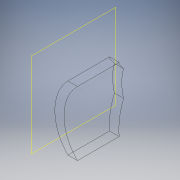
# Autodesk Inventor part: 14mm_radius_mold_with_crystal_skull
Saved by Autodesk Inventor 2018 (Build 220112000, 112)
## iProperties
Created: 2018-06-11
Part Number: 14mm_radius_mold_with_crystal_skull
Material: Generic
Document SubType Name: Modeling
Designer: McCormick Lab
Density: 1 g/cm^3
Appearance: Default
Author: McCormick Lab
Autodesk Inventor part; units mm, degrees
ref_plane "YZ Plane" through (0, 0, 0) normal (1, 0, 0) x (0, 1, 0)
ref_plane "XZ Plane" through (0, 0, 0) normal (0, 1, 0) x (-1, 0, 0)
ref_plane "XY Plane" through (0, 0, 0) normal (0, 0, 1) x (1, 0, 0)
sketch "Sketch1" plane through (0, 0, 0) normal (0, 1, 0) x (-1, 0, 0)
  arc A0 (0, -7) -> (0, 7) centre (0, 0) ccw
  line L0 (0, 7) -> (0, -7)
  dimension "d0" = 14
  constraints: 2 end point, 2 point on circle, 1 centre point, 1 coincident, 1 vertical
  measures "d0" diameter of A0
extrude "Extrusion1" add sketch "Sketch1" along normal blind 12
ref_plane "Work Plane1" through (-10, 0, 7) normal (1, 0, 0) x (0, 0, -1)
sketch "Sketch2" plane through (-10, 0, 7) normal (1, 0, 0) x (0, 0, -1)
  line L0 (2, 8) -> (2, 1.5)
  line L1 (2, 1.5) -> (12, 1.5)
  line L2 (12, 1.5) -> (12, 7.9943)
  line L3 (9, 10.4943) -> (5, 10.4943)
  line L4 (9, 10.4943) -> (12, 7.9943)
  line L5 (5, 10.4943) -> (2, 8)
  line L6 (14, 0) -> (14, 12) projected
  point P0 (7, 0)
  dimension "d9" = 10
  dimension "d10" = 6.5
  dimension "d12" = 4
  dimension "d14" = 3
  dimension "d15" = 3
  dimension "d24" = 2
  constraints: 12 end point, 1 horizontal, 1 parallel
  measures "d9" distance of L1.end L0.end
  measures "d10" distance of L0.end L0.start
  measures "d12" distance of L3.start L3.end
  measures "d14" horizontal distance of L0.end L3.end
  measures "d15" horizontal distance of L3.start L2.end
  measures "d24" distance between parallel lines of L6 L2
extrude "Extrusion2" add sketch "Sketch2" along normal blind 10
sketch "Sketch7" plane through (0, 0, 0) normal (0, 1, 0) x (-1, 0, 0)
  arc A0 (0, -7) -> (0, 7) centre (0, 0) ccw
  line L0 (0, 7) -> (0, -7)
  line L1 (0, -7) -> (0, 7)
  dimension "d40" = 7
  constraints: 4 end point, 2 point on circle, 1 centre point, 1 coincident, 1 collinear
  measures "d40" radius of A0
extrude "Extrusion7" cut sketch "Sketch7" along normal through all
sketch "Sketch9" plane through (0, 0, 0) normal (0, 1, 0) x (-1, 0, 0)
  arc A0 (6.399, -5) -> (6.399, 5) centre (1.2353, 0) ccw
  arc A1 (6.399, -5) -> (6.399, 5) centre (10.7308, 0) ccw
  point P0 (0, 0)
  constraints: 4 point on circle, 2 centre point
extrude "Extrusion9" cut sketch "Sketch9" along normal through all both and the other way through all
body "Solid1"
